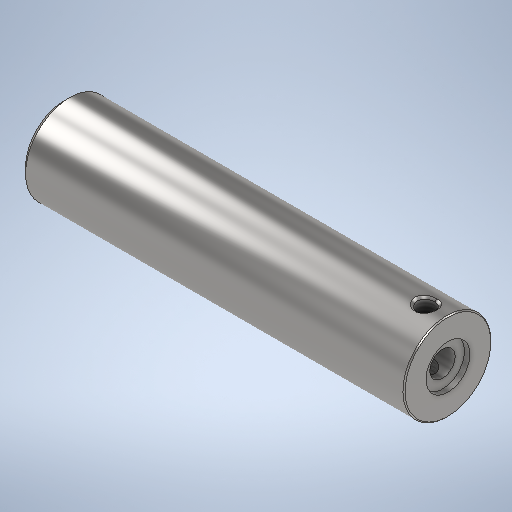
# Autodesk Inventor part: Sp mu SM holder
Saved by Autodesk Inventor 2026 (Build 300175050, 175E)
## iProperties
Created: 2025-06-20
Part Number: Sp mu SM holder
Material: Generic
Document SubType Name: Modeling
Designer: Annappa
Density: 1 g/cm^3
Appearance: Semi-Polished
Author: Annappa
Autodesk Inventor part; units mm, degrees
ref_plane "YZ Plane" through (0, 0, 0) normal (1, 0, 0) x (0, 1, 0)
ref_plane "XZ Plane" through (0, 0, 0) normal (0, 1, 0) x (-1, 0, 0)
ref_plane "XY Plane" through (0, 0, 0) normal (0, 0, 1) x (1, 0, 0)
sketch "Sketch1" plane through (0, 0, 0) normal (0, 0, 1) x (1, 0, 0)
  line L0 (0, 0) -> (0, 3)
  line L1 (0, 3) -> (15, 3)
  line L2 (15, 3) -> (15, 4)
  line L3 (15, 4) -> (35, 4)
  line L4 (35, 4) -> (35, 0)
  line L5 (35, 0) -> (0, 0)
  line L6 (34.5, 0) -> (34.5, 2)
  line L7 (34.5, 2) -> (35, 2)
  line L8 (34.5, 1.15) -> (31.5, 1.15)
  line L9 (31.5, 1.15) -> (30.7814, 0)
  line L10 (30.7814, 0) -> (34.5, 0)
  line L11 (15, 4) -> (0, 4)
  line L12 (0, 4) -> (0, 3)
  point P0 (0, 1.5)
  point P1 (35, 2)
  dimension "d0" = 3
  dimension "d1" = 4
  dimension "d2" = 15
  dimension "d3" = 35
  dimension "d4" = 2
  dimension "d5" = 0.5
  dimension "d27" = 1.15
  dimension "d28" = 58
  dimension "d29" = 3
  constraints: 26 end point, 6 perpendicular, 3 midpoint, 3 point on line, 2 collinear, 2 horizontal, 2 vertical
  measures "d0" distance between parallel lines of L1 L5
  measures "d1" distance from line of L0.start L3
  measures "d2" horizontal distance of L1.end point (0, 1.5)
  measures "d3" horizontal distance of L0.start point (35, 2)
  measures "d4" distance from line of L6.end L5
  measures "d5" distance between parallel lines of L6 L4
  measures "d27" distance between parallel lines of L8 L5
  measures "d28" angle of L8 L9
  measures "d29" distance of L8.start L8.end
revolve "Revolution1" add sketch "Sketch1" angle 360 about axis through (35, 0, 0) along (-1, 0, 0) contours L0 L1 L2 L3 L4 L7 L6 L8 L9 L5 | L12 L11 L2 L1
chamfer "Chamfer1" [suppressed]
chamfer "Chamfer2" distance 0.1 angle 45 1 edges at (35, -4, 0)
sketch "Sketch2" plane through (0, 0, 0) normal (0, 1, 0) x (-1, 0, 0)
  circle A0 centre (-33, 0) radius 0.8
  line L0 (-35, -2) -> (-35, 2) projected
  point P0 (0, 0)
  dimension "d13" = 1.6
  dimension "d14" = 2
  constraints: 1 centre point
  measures "d13" diameter of A0
  measures "d14" distance from line of A0.centre L0
extrude "Extrusion1" cut sketch "Sketch2" along normal mid plane 10
chamfer "Chamfer4" distance 0.2 angle 45 3 edges at (33, 3.9192, 0.8) (33.0001, 3.9192, -0.8) (33.8, -4, 0.001)
thread "Thread2" size "M1.6x0.35" class "6H" standard "ANSI Metric M Profile" length 5
thread "Thread3" size "M1.6x0.35" class "6H" standard "ANSI Metric M Profile" length 3
chamfer "Chamfer5" distance 0.5 angle 45 1 edges at (0, -4, 0)
body "Solid1"
